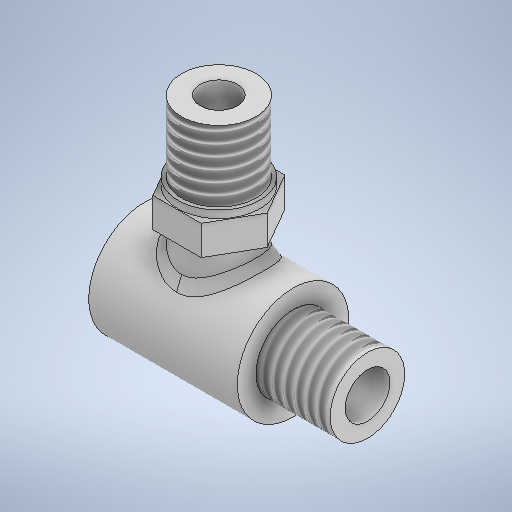
# Autodesk Inventor part: 123
Saved by Autodesk Inventor 2025.1 (Build 291241000, 241)
## iProperties
Created: 2024-08-21
Part Number: 123
Material: Generisch
Document SubType Name: Modeling
Designer: ffogue
Density: 1 g/cm^3
Appearance: Vorgabe
Author: ffogue
Autodesk Inventor part; units mm, degrees
ref_plane "YZ Plane" through (0, 0, 0) normal (1, 0, 0) x (0, 1, 0)
sketch "Sketch1" plane through (0, 0, 0) normal (0, 0, 1) x (1, 0, 0)
  line L0 (0, 0) -> (0, 7.5)
  line L1 (0, 7.5) -> (20, 7.5)
  line L2 (20, 7.5) -> (20, 5)
  line L3 (20, 5) -> (30, 5)
  line L4 (30, 5) -> (30, 0)
  line L5 (30, 0) -> (0, 0)
  dimension "d0" = 30
  dimension "d1" = 10
  dimension "d2" = 15
  dimension "d3" = 10
  constraints: 12 end point, 5 perpendicular, 1 vertical
  measures "d0" distance between parallel lines of L4 L0
  measures "d1" distance of L2.end L3.end
  measures "d2" diameter of L1 L5
  measures "d3" diameter of L3 L5
revolve "Revolution1" add sketch "Sketch1" angle 360 about axis through (30, 0, 0) along (-1, 0, 0)
ref_plane "Work Plane1" through (0, 0, 25) normal (0, 0, 1) x (1, 0, 0)
sketch "Sketch2" plane through (0, 0, 25) normal (0, 0, 1) x (1, 0, 0)
  circle A0 centre (10, 0) radius 5
  point P0 (0, 0)
  dimension "d6" = 10
  dimension "d7" = 10
  constraints: 1 centre point, 1 horizontal alignment
  measures "d6" diameter of A0
  measures "d7" distance of point (0, 0) A0.centre
extrude "Extrusion1" add sketch "Sketch2" against normal up to surface
ref_plane "Work Plane2" through (0, 0, 12.5) normal (0, 0, 1) x (1, 0, 0)
sketch "Sketch3" plane through (0, 0, 12.5) normal (0, 0, 1) x (1, 0, 0)
  spline S0 degree 5 poles (15, 0) (15, 0.4219) (14.9555, 0.8387) (14.8687, 1.2398) (14.7463, 1.6158) (14.3477, 2.5523) (14.0183, 3.0596) (13.6471, 3.4841) (13.2419, 3.8427) (12.55, 4.312) (12.2828, 4.4645) (12.0061, 4.5954) (11.7208, 4.7045) (11.1518, 4.8741) (10.869, 4.9367) (10.5813, 4.9788) (10.2907, 5) (9.7153, 5) (9.4311, 4.9798) (9.1493, 4.9393) (8.8717, 4.8792) (8.3043, 4.7138) (8.0156, 4.6048) (7.7353, 4.4738) (7.4645, 4.3208) (6.884, 3.9294) (6.5801, 3.6794) (6.2931, 3.3932) (6.0271, 3.0673) (5.633, 2.4524) (5.4882, 2.1871) (5.3591, 1.9015) (5.2496, 1.5959) (5.0609, 0.8779) (4.9924, 0.4546) (4.9713, 0.0174) (4.9997, -0.4169) (5.1096, -1.0686) (5.1632, -1.2988) (5.2289, -1.5209) (5.305, -1.7336) (5.509, -2.2194) (5.6454, -2.4831) (5.7955, -2.7277) (5.957, -2.9541) (6.3184, -3.3966) (6.521, -3.6087) (6.7335, -3.8013) (6.9549, -3.9755) (7.4457, -4.3099) (7.7178, -4.4651) (7.9996, -4.5981) (8.29, -4.7088) (8.8615, -4.877) (9.1415, -4.9382) (9.4259, -4.9794) (9.7127, -5) (10.2898, -5) (10.5796, -4.979) (10.8666, -4.9371) (11.1485, -4.8748) (11.7152, -4.7064) (11.9989, -4.5984) (12.2741, -4.4688) (12.5399, -4.3179) (13.116, -3.9294) (13.4199, -3.6794) (13.7069, -3.3932) (13.973, -3.0673) (14.367, -2.4524) (14.5118, -2.1871) (14.6409, -1.9015) (14.7504, -1.5959) (14.8987, -1.0314) (14.9486, -0.7812) (14.9828, -0.5236) (15, -0.2621) (15, 0) knots 0 0 0 0 0 0 0.052953 0.052953 0.052953 0.052953 0.144858 0.144858 0.144858 0.144858 0.19905 0.19905 0.19905 0.19905 0.250146 0.250146 0.250146 0.250146 0.300195 0.300195 0.300195 0.300195 0.355044 0.355044 0.355044 0.355044 0.42274 0.42274 0.42274 0.42274 0.467615 0.467615 0.467615 0.467615 0.521968 0.521968 0.521968 0.521968 0.553072 0.553072 0.553072 0.553072 0.596617 0.596617 0.596617 0.596617 0.645101 0.645101 0.645101 0.645101 0.700146 0.700146 0.700146 0.700146 0.75049 0.75049 0.75049 0.75049 0.801269 0.801269 0.801269 0.801269 0.854949 0.854949 0.854949 0.854949 0.922334 0.922334 0.922334 0.922334 0.967006 0.967006 0.967006 0.967006 1 1 1 1 1 1 projected
  line L0 (0, 7.5) -> (0, -7.5) projected
  line L1 (20, 7.5) -> (20, -7.5) projected
  line L2 (3.5, 0) -> (6.75, 5.6292)
  line L3 (6.75, 5.6292) -> (13.25, 5.6292)
  line L4 (13.25, 5.6292) -> (16.5, 0)
  line L5 (16.5, 0) -> (13.25, -5.6292)
  line L6 (13.25, -5.6292) -> (6.75, -5.6292)
  line L7 (6.75, -5.6292) -> (3.5, 0)
  point P0 (0, 0)
  point P1 (10, 0)
  dimension "d11" = 13
  dimension "d12" = 10
  constraints: 12 end point, 1 horizontal alignment, 14 other
  measures "d11" distance of L4.end L2.start
  measures "d12" distance from line of L0 point (10, 0)
extrude "Extrusion2" add sketch "Sketch3" along normal mid plane 4
chamfer "Chamfer1" distance 1 angle 45 1 edges at (5.0001, 0.0275, 7.4999)
sketch "Sketch4" plane through (10, 0, 25) normal (0, 0, 1) x (1, 0, 0)
  circle A0 centre (0, 0) radius 5 projected
  point P0 (-10, 0)
  constraints: 1 coincident
hole "Hole1" at (10, 0, 25) direction (0, 0, -1) diameter 5 depth 25
sketch "Sketch5" plane through (0, 0, 0) normal (-1, 0, 0) x (0, 0, 1)
  circle A0 centre (0, 0) radius 7.5 projected
  constraints: 1 coincident
hole "Hole2" at (0, 0, 0) direction (1, 0, 0) diameter 8 depth 16
sketch "Sketch6" plane through (30, 0, 0) normal (1, 0, 0) x (0, 0, -1)
  circle A0 centre (0, 0) radius 5 projected
  constraints: 1 coincident
hole "Hole3" at (30, 0, 0) direction (-1, 0, 0) diameter 6 depth 14
thread "Thread2" size "M8x1.25" class "6H" standard "ISO Metric profile" length 9
sketch "Sketch7" plane through (0, 0, 14.5) normal (0, 0, 1) x (1, 0, 0)
  circle A0 centre (10, 0) radius 2.5 projected
  line L0 (6.75, -5.6292) -> (3.5, 0) projected
  line L1 (3.5, 0) -> (6.75, 5.6292) projected
  line L2 (6.75, 5.6292) -> (13.25, 5.6292) projected
  line L3 (13.25, 5.6292) -> (16.5, 0) projected
  line L4 (16.5, 0) -> (13.25, -5.6292) projected
  line L5 (13.25, -5.6292) -> (6.75, -5.6292) projected
  circle A1 centre (10, 0) radius 5 projected
  circle A2 centre (10, 0) radius 5.5
  point P0 (0, 0)
  dimension "d43" = 11
  constraints: 1 centre point, 1 coincident
  measures "d43" diameter of A2
extrude "Extrusion3" add sketch "Sketch7" along normal blind 1 contours A2
thread "Thread3" size "M10x1.5" class "6g" standard "ISO Metric profile" length 9.5
thread "Thread4" size "M10x1.5" class "6g" standard "ISO Metric profile" length 9.5
body "Solid1"
